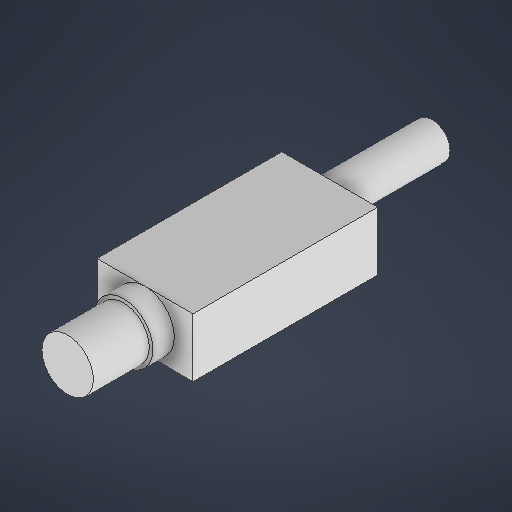
# Autodesk Inventor part: Updated Laser Scanner
Saved by Autodesk Inventor 2025 (Build 290162000, 162)
## iProperties
Created: 2024-04-26
Part Number: Updated Laser Scanner
Material: Generic
Document SubType Name: Modeling
Designer: Thienan Hoang
Density: 1 g/cm^3
Appearance: Default
Author: Thienan Hoang
Autodesk Inventor part; units mm, degrees
ref_plane "YZ Plane" through (0, 0, 0) normal (1, 0, 0) x (0, 1, 0)
ref_plane "XZ Plane" through (0, 0, 0) normal (0, 1, 0) x (-1, 0, 0)
ref_plane "XY Plane" through (0, 0, 0) normal (0, 0, 1) x (1, 0, 0)
sketch "Sketch1" plane through (0, 0, 0) normal (0, 1, 0) x (-1, 0, 0)
  line L0 (33.5, 64.5) -> (-33.5, 64.5)
  line L1 (-33.5, 64.5) -> (-33.5, -64.5)
  line L2 (-33.5, -64.5) -> (33.5, -64.5)
  line L3 (33.5, -64.5) -> (33.5, 64.5)
  line L4 (33.5, 64.5) -> (-33.5, -64.5) construction
  line L5 (-33.5, 64.5) -> (33.5, -64.5) construction
  point P0 (0, 0)
  dimension "d0" = 67
  dimension "d1" = 129
  constraints: 12 end point, 2 midpoint, 2 parallel, 1 horizontal, 1 perpendicular
  measures "d0" distance of L2.end L1.end
  measures "d1" distance of L1.end L0.end
extrude "Extrusion1" add sketch "Sketch1" along normal blind 41
sketch "Sketch2" plane through (-33.5, 0, 64.5) normal (0, 0, 1) x (1, 0, 0)
  circle A0 centre (33.5, 20.5) radius 20.5
  circle A1 centre (33.5, 20.5) radius 18
  point P0 (33.5, 0)
  dimension "d4" = 41
  dimension "d5" = 36
  constraints: 2 centre point, 1 coincident
  measures "d4" diameter of A0
  measures "d5" diameter of A1
extrude "Extrusion2" add sketch "Sketch2" along normal blind 54 contours A1
extrude "Extrusion3" add sketch "Sketch2" along normal blind 15
sketch "Sketch4" plane through (33.5, 0, -64.5) normal (0, 0, -1) x (-1, 0, 0)
  circle A0 centre (42, 20.5) radius 12.5
  line L0 (67, 0) -> (67, 41) projected
  point P0 (33.5, 0)
  dimension "d13" = 25
  dimension "d14" = 25
  constraints: 1 centre point
  measures "d13" diameter of A0
  measures "d14" distance from line of L0 A0.centre
extrude "Extrusion5" add sketch "Sketch4" along normal blind 80
sketch "Sketch5" plane through (0, 0, 0) normal (0, -1, 0) x (1, 0, 0)
  circle A0 centre (0, 51.5) radius 2.5
  circle A1 centre (0, 8.5) radius 2.5
  circle A2 centre (0, -21.5) radius 2
  circle A3 centre (0, -33.5) radius 2.5
  line L0 (-2, 39.5) -> (-2, 37.5)
  line L1 (2, 37.5) -> (2, 39.5)
  arc A4 (2, 39.5) -> (-2, 39.5) centre (0, 39.5) ccw
  arc A5 (-2, 37.5) -> (2, 37.5) centre (0, 37.5) ccw
  line L2 (18, 118.5) -> (-18, 118.5) projected
  point P0 (2, 38.5)
  point P1 (-2, 38.5)
  dimension "d17" = 5
  dimension "d19" = 4
  dimension "d20" = 5
  dimension "d23" = 67
  dimension "d24" = 80
  dimension "d25" = 110
  dimension "d35" = 85
  dimension "d36" = 60
  constraints: 6 centre point, 4 end point, 4 point on circle, 2 midpoint, 1 coincident, 1 parallel
  measures "d17" diameter of A0
  measures "d19" diameter of A2
  measures "d20" diameter of A3
  measures "d23" distance from line of L2 A0.centre
  measures "d24" distance from line of L2 point (2, 38.5)
  measures "d25" distance from line of L2 A1.centre
  measures "d35" distance of A3.centre A0.centre
  measures "d36" vertical distance of A2.centre point (-2, 38.5)
hole "Hole1" at (0, 0, 51.5) at (0, 0, -33.5) direction (0, 1, 0) diameter 4.917 depth 10 thread size "M6x1" class "6H" standard "ANSI Metric M Profile"
hole "Hole2" at (0, 0, 8.5) direction (0, 1, 0) diameter 4.9784 depth 10 thread size "1/4-20 UNC" class "2B" standard "ANSI Unified Screw Threads"
hole "Hole3" at (0, 0, 39.5) at (0, 0, 37.5) at (0, 0, -21.5) direction (0, 1, 0) diameter 4 depth 10
body "Solid1"
